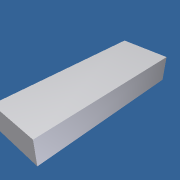
# Autodesk Inventor part: Box
Saved by Autodesk Inventor 2012 (Build 160160000, 160)
## iProperties
Created: 2009-08-07
Part Number: Box
Document SubType Name: Modeling
Designer: leefsmp
Density: 1 g/cm^3
Mass: 12 g
Surface Area: 40 cm^2
Volume: 12 cm^3
Material: Default
Author: leefsmp
Autodesk Inventor part; units mm, degrees
ref_plane "YZ Plane" through (0, 0, 0) normal (1, 0, 0) x (0, 1, 0)
ref_plane "XZ Plane" through (0, 0, 0) normal (0, 1, 0) x (-1, 0, 0)
ref_plane "XY Plane" through (0, 0, 0) normal (0, 0, 1) x (1, 0, 0)
sketch "Sketch1" plane through (0, 0, 0) normal (0, 0, 1) x (1, 0, 0)
  line L0 (-10, -30) -> (10, -30)
  line L1 (10, -30) -> (10, 30)
  line L2 (10, 30) -> (-10, 30)
  line L3 (-10, 30) -> (-10, -30)
  point P0 (0, 0)
  dimension "y1" = 30
  dimension "y2" = 30
  dimension "x1" = 10
  dimension "x2" = 10
  constraints: 8 end point, 2 parallel, 1 horizontal, 1 perpendicular
  measures "y1" distance from line of L2 point (0, 0)
  measures "y2" distance from line of L0 point (0, 0)
  measures "x1" distance from line of L1 point (0, 0)
  measures "x2" distance from line of L3 point (0, 0)
extrude "Extrusion1" add sketch "Sketch1" along normal mid plane 10
equation "\"y1\" = 0.5 * y"
equation "\"y2\" = 0.5 * y"
equation "\"x1\" = 0.5 * x"
equation "\"x2\" = 0.5 * x"
equation "\"z2\" = z"
equation "\"z\" = 10"
equation "\"y\" = 60"
equation "\"x\" = 20"
body "Solid1"
